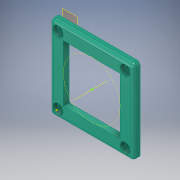
# Autodesk Inventor part: 10_Lid_1x1_v2_thin
Saved by Autodesk Inventor 2019 (Build 230136000, 136)
## iProperties
Created: 2019-07-01
Part Number: 10_Lid_1x1_v2_thin
Material: Generic
Document SubType Name: Modeling
Designer: diederichbenedict
Density: 1 g/cm^3
Appearance: IPHT_Türkis
Author: diederichbenedict
Autodesk Inventor part; units mm, degrees
ref_plane "YZ Plane" through (0, 0, 0) normal (1, 0, 0) x (0, 1, 0)
ref_plane "XZ Plane" through (0, 0, 0) normal (0, 1, 0) x (-1, 0, 0)
ref_plane "XY Plane" through (0, 0, 0) normal (0, 0, 1) x (1, 0, 0)
ref_plane "Work Plane1" through (0, 41.8, 0) normal (0, 0, 1) x (1, 0, 0)
sketch "Sketch1" plane through (0, 41.8, 0) normal (0, 0, 1) x (1, 0, 0)
  line L0 (4, 0.3838) -> (4, 4) construction
  line L1 (4, 4) -> (-2, 4) construction
  arc A0 (-2, 4) -> (-4, 2) centre (-2, 2) ccw construction
  line L2 (-4, 2) -> (-4, -4) construction
  line L3 (-4, -4) -> (-0.3838, -4) construction
  arc A1 (45.8, 2) -> (43.8, 4) centre (43.8, 2) ccw construction
  line L4 (43.8, 4) -> (37.8, 4) construction
  line L5 (37.8, 4) -> (37.8, 0.3838) construction
  line L6 (42.1838, -4) -> (45.8, -4) construction
  line L7 (45.8, -4) -> (45.8, 2) construction
  line L8 (37.8, -42.1838) -> (37.8, -45.8) construction
  line L9 (37.8, -45.8) -> (43.8, -45.8) construction
  arc A2 (43.8, -45.8) -> (45.8, -43.8) centre (43.8, -43.8) ccw construction
  line L10 (45.8, -43.8) -> (45.8, -37.8) construction
  line L11 (45.8, -37.8) -> (42.1838, -37.8) construction
  line L12 (-0.3838, -37.8) -> (-4, -37.8) construction
  line L13 (-4, -37.8) -> (-4, -43.8) construction
  arc A3 (-4, -43.8) -> (-2, -45.8) centre (-2, -43.8) ccw construction
  line L14 (-2, -45.8) -> (4, -45.8) construction
  line L15 (4, -45.8) -> (4, -42.1838) construction
  line L16 (-2, 4) -> (43.8, 4)
  line L17 (45.8, 2) -> (45.8, -43.8)
  line L18 (43.8, -45.8) -> (-2, -45.8)
  line L19 (-4, -43.8) -> (-4, 2)
  line L20 (40.3, -37.8) -> (40.3, -4)
  line L21 (37.8, -1.5) -> (4, -1.5)
  line L22 (1.5, -4) -> (1.5, -37.8)
  line L23 (4, -40.3) -> (37.8, -40.3)
  line L24 (37.8, -40.3) -> (40.3, -37.8)
  line L25 (4, -40.3) -> (1.5, -37.8)
  line L26 (4, -1.5) -> (1.5, -4)
  line L27 (40.3, -4) -> (37.8, -1.5)
  arc A4 (45.8, 2) -> (43.8, 4) centre (43.8, 2) ccw
  arc A5 (43.8, -45.8) -> (45.8, -43.8) centre (43.8, -43.8) ccw
  arc A6 (-4, -43.8) -> (-2, -45.8) centre (-2, -43.8) ccw
  arc A7 (-2, 4) -> (-4, 2) centre (-2, 2) ccw
  circle A8 centre (1, -1) radius 1.4
  circle A9 centre (40.8, -1) radius 1.4
  circle A10 centre (40.8, -40.8) radius 1.4
  circle A11 centre (1, -40.8) radius 1.4
  circle A12 centre (20.9, -20.9) radius 19.4 construction
  line L28 (4, -4) -> (4, -37.8)
  line L29 (4, -37.8) -> (37.8, -37.8)
  line L30 (37.8, -37.8) -> (37.8, -4)
  line L31 (37.8, -4) -> (4, -4)
  arc A13 (39.5978, -40.386) -> (40.386, -39.5978) centre (40.9, -40.9) ccw projected
  line L32 (39.5978, -40.386) -> (37.8, -42.1838) projected
  line L33 (42.1838, -37.8) -> (40.386, -39.5978) projected
  arc A14 (1.414, -39.5978) -> (2.2022, -40.386) centre (0.9, -40.9) ccw projected
  line L34 (1.414, -39.5978) -> (-0.3838, -37.8) projected
  line L35 (4, -42.1838) -> (2.2022, -40.386) projected
  arc A15 (40.386, -2.2022) -> (39.5978, -1.414) centre (40.9, -0.9) ccw projected
  line L36 (40.386, -2.2022) -> (42.1838, -4) projected
  line L37 (37.8, 0.3838) -> (39.5978, -1.414) projected
  arc A16 (2.2022, -1.414) -> (1.414, -2.2022) centre (0.9, -0.9) ccw projected
  line L38 (2.2022, -1.414) -> (4, 0.3838) projected
  line L39 (-0.3838, -4) -> (1.414, -2.2022) projected
  point P0 (45.8, -45.8)
  point P1 (45.8, 4)
  point P2 (-4, -45.8)
  point P3 (40.3, -40.3)
  point P4 (40.3, -1.5)
  point P5 (1.5, -1.5)
  point P6 (1.5, -40.3)
  point P7 (40.8, -1)
  dimension "d55" = 2.8
  dimension "d56" = 2.8
  dimension "d57" = 2.8
  dimension "d58" = 2.8
  dimension "d34" = 49.8
  dimension "d35" = 49.8
  dimension "d36" = 5.5
  dimension "d37" = 2.5
  dimension "d38" = 2.5
  dimension "d39" = 2.5
  dimension "d40" = 2.5
  dimension "d41" = 2.5
  dimension "d42" = 2.5
  dimension "d43" = 2.5
  dimension "d44" = 2.5
  dimension "d45" = 2
  dimension "d46" = 5
  dimension "d47" = 5
  dimension "d48" = 5
  dimension "d49" = 5
  dimension "d50" = 5
  dimension "d51" = 5
  dimension "d52" = 0.5
  dimension "d53" = 5
  dimension "d54" = 5
  dimension "d90" = 8
  constraints: 32 end point, 14 point on line, 11 tangent, 8 point on circle, 6 parallel, 5 centre point, 3 coincident, 3 equal radius, 3 perpendicular, 1 horizontal, 14 other
  measures "d34" distance of point (45.8, -45.8) point (-4, -45.8)
  measures "d35" distance of point (45.8, 4) point (45.8, -45.8)
  measures "d36" distance between parallel lines of L17 L20
  measures "d37" distance of L23.end point (40.3, -40.3)
  measures "d38" distance of L20.start point (40.3, -40.3)
  measures "d39" distance of L23.start point (1.5, -40.3)
  measures "d40" distance of L22.end point (1.5, -40.3)
  measures "d41" distance of L21.end point (1.5, -1.5)
  measures "d42" distance of L22.start point (1.5, -1.5)
  measures "d43" distance of L20.end point (40.3, -1.5)
  measures "d44" distance of L21.start point (40.3, -1.5)
  measures "d45" radius of A4
  measures "d46" distance from line of point (1, -40.8) L19
  measures "d47" distance from line of L18 point (1, -40.8)
  measures "d48" distance from line of L17 point (40.8, -40.8)
  measures "d49" distance from line of L18 point (40.8, -40.8)
  measures "d50" distance from line of L7 point (40.8, -1)
  measures "d51" distance from line of L16 point (40.8, -1)
  measures "d52" distance from line of point (1, -1) L22
  measures "d53" distance from line of L2 point (1, -1)
  measures "d54" distance from line of L1 point (1, -1)
  measures "d90" distance between parallel lines of L19 L28
extrude "Extrusion1" add sketch "Sketch1" along normal blind 8 contours L16 A4 L17 A5 L18 A6 L19 A7 | L24 L23 L25 L22 L26 L21 L27 L20 | A8 A16 | A9 A15 | A10 A13 | A14 A11
fillet "Fillet1" radius 2 8 edges at (20.9, -4, 8) (45.2142, -3.4142, 8) (45.8, 20.9, 8) (45.2142, 45.2142, 8) (20.9, 45.8, 8) (-3.4142, 45.2142, 8) (-4, 20.9, 8) (-3.4142, -3.4142, 8)
sketch "Sketch2" plane through (-2, -4, 0) normal (0, -1, 0) x (1, 0, 0)
  line L0 (43.8, -4.8712) -> (42.35, -4)
  line L1 (2, -4.8712) -> (0.55, -4)
  line L2 (-2, 0) -> (-2, 6) construction
  line L3 (45.8, 8) -> (0, 8) construction
  line L4 (47.8, 0) -> (47.8, 6) construction
  circle A0 centre (2.9, -36.9) radius 1.45 projected
  line L5 (0, -41.8) -> (45.8, -41.8) projected
  point P0 (2, 0)
  point P1 (2.9, 3.1)
  point P2 (42.9, 3.1)
  dimension "d59" = 4.9
  dimension "d60" = 4.9
  dimension "d61" = 4.9
  dimension "d62" = 4.9
  constraints: 4 end point, 6 other
  measures "d59" distance from line of point (2.9, 3.1) L2
  measures "d60" distance from line of point (2.9, 3.1) L3
  measures "d61" distance from line of point (42.9, 3.1) L4
  measures "d62" distance from line of point (42.9, 3.1) L3
hole "Hole1" [suppressed]
sketch "Sketch3" plane through (0, 41.8, 8) normal (0, 0, 1) x (1, 0, 0)
  circle A0 centre (20.9, -20.9) radius 16.9 construction
  point P0 (0, -41.8)
  constraints: 1 centre point
sketch "Sketch4" plane through (0, 41.8, 8) normal (0, 0, 1) x (1, 0, 0)
  line L0 (37.8, -37.8) -> (37.8, -4) projected
  line L1 (37.8, -4) -> (4, -4) projected
  line L2 (4, -4) -> (4, -37.8) projected
  line L3 (4, -37.8) -> (37.8, -37.8) projected
  circle A0 centre (40.9, -0.9) radius 2.75 projected
  circle A1 centre (0.9, -40.9) radius 2.75 projected
  circle A2 centre (0.9, -0.9) radius 2.75 projected
  circle A3 centre (40.9, -40.9) radius 2.75 projected
  line L4 (43.8, 2) -> (-2, 2) projected
  line L5 (43.8, -43.8) -> (43.8, 2) projected
  line L6 (-2, -43.8) -> (43.8, -43.8) projected
  line L7 (-2, 2) -> (-2, -43.8) projected
hole "Hole2" at (40.9, 40.9, 8) at (40.9, 0.9, 8) at (0.9, 0.9, 8) at (0.9, 40.9, 8) direction (0, 0, -1) diameter 3.2 depth 12 tip angle 118 counterbore diameter 6 counterbore depth 2.5
chamfer "Chamfer2" distance 4.5 angle 45 2 edges at (4, 20.9, 0) (37.8, 20.9, 0)
sketch "Sketch6" plane through (-4, -2, 0) normal (-1, 0, 0) x (0, 0, 1)
  line L0 (0, -2) -> (6, -2) construction
  line L1 (8, 0) -> (8, 45.8) construction
  line L2 (0, 47.8) -> (6, 47.8) construction
  circle A0 centre (3.1, 42.9) radius 1.4 construction
  circle A1 centre (3.1, 2.9) radius 1.4 construction
  point P0 (0, 2)
  dimension "d63" = 2.8
  dimension "d64" = 2.8
  dimension "d65" = 4.9
  dimension "d66" = 4.9
  dimension "d67" = 4.9
  dimension "d68" = 4.9
  constraints: 2 centre point
  measures "d63" diameter of A0
  measures "d64" diameter of A1
  measures "d65" distance from line of A0.centre L1
  measures "d66" distance from line of A0.centre L2
  measures "d67" distance from line of A1.centre L0
  measures "d68" distance from line of L1 A1.centre
hole "Hole3" [suppressed]
sketch "Sketch7" plane through (45.8, -2, 0) normal (1, 0, 0) x (0, 0, -1)
  circle A0 centre (-3.1, 42.9) radius 1.4 projected
  circle A1 centre (-3.1, 2.9) radius 1.4 projected
  point P0 (0, 2)
hole "Hole4" [suppressed]
sketch "Sketch8" plane through (-2, 45.8, 0) normal (0, 1, 0) x (1, 0, 0)
  circle A0 centre (2.9, -3.1) radius 1.45 projected
  circle A1 centre (42.9, -3.1) radius 1.45 projected
  point P0 (2, 0)
  point P1 (4.35, -3.1)
  point P2 (4.35, -3.1)
  point P3 (44.35, -3.1)
  point P4 (44.35, -3.1)
hole "Hole5" [suppressed]
sketch "Sketch9" plane through (37.8, 4, 8) normal (-1, 0, 0) x (0, 0, 1)
  line L0 (-8, 0) -> (-3.5, 0) projected
  line L1 (-3.5, 33.8) -> (-8, 33.8) projected
  line L2 (-3.5, 0) -> (-8, -4.5)
  line L3 (-8, 39.8) -> (-8, -6) projected
  line L4 (-3.5, 0) -> (2.864, 0) construction
  line L5 (-8, -4.5) -> (-8, 0)
  line L6 (-3.5, 33.8) -> (-8, 38.3)
  line L7 (-3.5, 33.8) -> (2.864, 33.8) construction
  line L8 (-8, 38.3) -> (-8, 33.8)
  line L9 (-8, 33.8) -> (-3.5, 33.8)
  point P0 (-8, -4)
  dimension "d91" = 135
  dimension "d92" = 135
  constraints: 14 end point, 3 collinear, 2 equal length, 2 horizontal, 2 point on line
  measures "d91" angle of L2 L4
  measures "d92" angle of L7 L6
extrude "Extrusion3" cut sketch "Sketch9" along normal up to surface (33.8 mm away)
sketch "Sketch13" plane through (0, 41.8, 0) normal (0, 0, -1) x (-1, 0, 0)
  line L0 (-37.8, -42.3) -> (-37.8, -37.8) projected
  line L1 (-37.8, -37.8) -> (-42.3, -37.8) projected
  line L2 (-42.3, -4) -> (-42.3, -37.8) projected
  line L3 (-42.3, -4) -> (-37.8, -4) projected
  line L4 (-37.8, -4) -> (-37.8, 0.5) projected
  line L5 (-37.8, 0.5) -> (-4, 0.5) projected
  line L6 (-4, 0.5) -> (-4, -4) projected
  line L7 (-4, -4) -> (0.5, -4) projected
  line L8 (0.5, -37.8) -> (0.5, -4) projected
  line L9 (0.5, -37.8) -> (-4, -37.8) projected
  line L10 (-4, -37.8) -> (-4, -42.3) projected
  line L11 (-4, -42.3) -> (-37.8, -42.3) projected
  circle A0 centre (-0.9, -40.9) radius 1.6 projected
  circle A1 centre (-40.9, -0.9) radius 1.6 projected
  circle A2 centre (-40.9, -40.9) radius 1.6 projected
  circle A3 centre (-0.9, -0.9) radius 1.6 projected
  line L12 (-45.8, 2) -> (-45.8, -43.8) projected
  arc A4 (-45.8, -43.8) -> (-43.8, -45.8) centre (-43.8, -43.8) ccw projected
  line L13 (-43.8, -45.8) -> (2, -45.8) projected
  arc A5 (2, -45.8) -> (4, -43.8) centre (2, -43.8) ccw projected
  line L14 (4, -43.8) -> (4, 2) projected
  arc A6 (4, 2) -> (2, 4) centre (2, 2) ccw projected
  line L15 (2, 4) -> (-43.8, 4) projected
  arc A7 (-43.8, 4) -> (-45.8, 2) centre (-43.8, 2) ccw projected
  point P0 (0, -41.8)
extrude "Extrusion5" cut sketch "Sketch13" against normal blind 4 contours L0 L1 L2 L3 L4 L5 L6 L7 L8 L9 L10 L11 | A7 L15 A6 L14 A5 L13 A4 L12
equation "\"d38\" = d37"
equation "\"d39\" = d37"
equation "\"d40\" = d39"
equation "\"d41\" = d37"
equation "\"d42\" = d41"
equation "\"d43\" = d37"
equation "\"d44\" = d43"
body "Solid1"
